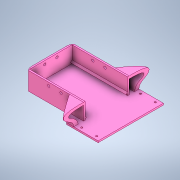
# Autodesk Inventor part: Body_001
Saved by Autodesk Inventor 2021 (Build 250183000, 183)
## iProperties
Created: 2022-04-07
Part Number: Body_001
Material: Genérico
Document SubType Name: Modeling
Designer: skatl
Density: 1 g/cm^3
Appearance: Rosado
Author: skatl
Autodesk Inventor part; units mm, degrees
ref_plane "YZ Plane" through (0, 0, 0) normal (1, 0, 0) x (0, 1, 0)
ref_plane "XZ Plane" through (0, 0, 0) normal (0, 1, 0) x (-1, 0, 0)
ref_plane "XY Plane" through (0, 0, 0) normal (0, 0, 1) x (1, 0, 0)
sketch "Boceto1" plane through (0, 0, 0) normal (0, 1, 0) x (-1, 0, 0)
  line L0 (-50, -35) -> (50, -35)
  line L1 (50, -35) -> (50, 35)
  line L2 (50, 35) -> (-50, 35)
  line L3 (-50, 35) -> (-50, -35)
  line L4 (-50, -35) -> (50, 35) construction
  line L5 (50, -35) -> (-50, 35) construction
  line L6 (-50, -35) -> (-20, -35)
  line L7 (-20, -35) -> (-20, 35)
  line L8 (-20, 35) -> (-50, 35)
  line L9 (-50, 35) -> (-50, -35)
  line L10 (-20, 40) -> (-50, 40)
  line L11 (-50, 40) -> (-50, -40)
  line L12 (-50, -40) -> (-20, -40)
  line L13 (-20, -40) -> (-20, 40)
  line L14 (-20, 40) -> (-50, -40) construction
  line L15 (-50, 40) -> (-20, -40) construction
  point P0 (0, 0)
  point P1 (-35, 0)
  dimension "d0" = 100
  dimension "d1" = 70
  dimension "d67" = 30
  dimension "d68" = 30
  dimension "d69" = 80
  constraints: 32 end point, 6 parallel, 4 midpoint, 3 horizontal, 3 perpendicular, 1 point on line
  measures "d0" distance of L2.end L1.end
  measures "d1" distance of L1.end L0.end
  measures "d67" distance of L8.end L7.end
  measures "d68" distance of L12.end L11.end
  measures "d69" distance of L11.end L10.end
extrude "Extrusión1" add sketch "Boceto1" along normal blind 22 contours L3 L2 L7 L0 | L7 L2 L1 L0
sketch "Boceto2" plane through (-50, 0, 35) normal (0, 0, 1) x (1, 0, 0)
  line L0 (0, 0) -> (100, 0) projected
  line L1 (100, 0) -> (70, 0)
  line L2 (70, 0) -> (70, 2)
  line L3 (70, 2) -> (100, 2)
  line L4 (100, 2) -> (100, 0)
  line L5 (0, 22) -> (100, 22) projected
  line L6 (70, 2) -> (100, 2)
  line L7 (100, 2) -> (100, 22)
  line L8 (100, 22) -> (70, 22)
  line L9 (70, 22) -> (70, 2)
  point P0 (50, 0)
  point P1 (70, 22)
  dimension "d4" = 30
  dimension "d5" = 2
  constraints: 16 end point, 4 parallel, 2 horizontal, 2 perpendicular
  measures "d4" distance of L2.end L3.end
  measures "d5" distance of L1.end L2.end
extrude "Extrusión2" cut sketch "Boceto2" against normal through all contours L9 L5 L7 L3
sketch "Boceto3" plane through (-50, 0, 35) normal (0, 0, 1) x (1, 0, 0)
  line L0 (70, 22) -> (0, 22) projected
  line L1 (35, 22) -> (35, 0)
  line L2 (70, 2) -> (70, 22) projected
  line L3 (70, 12) -> (-10, 12)
  line L4 (27.5, 3) -> (42.5, 3)
  line L5 (42.5, 3) -> (42.5, 21)
  line L6 (42.5, 21) -> (27.5, 21)
  line L7 (27.5, 21) -> (27.5, 3)
  line L8 (27.5, 3) -> (42.5, 21) construction
  line L9 (42.5, 3) -> (27.5, 21) construction
  line L10 (42.5, 21) -> (42.5, 18)
  circle A0 centre (42.5, 18) radius 1.5
  circle A1 centre (27.5, 18) radius 1.5
  point P0 (50, 0)
  point P1 (35, 12)
  dimension "d31" = 15
  dimension "d32" = 18
  dimension "d33" = 3
  dimension "d34" = 3
  constraints: 18 end point, 4 midpoint, 3 point on line, 2 centre point, 2 coincident, 2 horizontal, 2 parallel, 2 symmetric about line, 1 perpendicular, 1 vertical, 1 other
  measures "d31" distance of L6.end L5.end
  measures "d32" distance of L5.end L4.end
  measures "d33" distance of L5.end L10.end
  measures "d34" diameter of A0
extrude "Extrusión3" cut sketch "Boceto3" against normal through all contours A0 L5 | L5 A0 | A1 L7 | L7 A1
sketch "Boceto4" plane through (-50, 0, -35) normal (-1, 0, 0) x (0, 0, 1)
  line L0 (35, 22) -> (35, 0)
  line L1 (27.5, 3) -> (42.5, 3)
  line L2 (42.5, 3) -> (42.5, 21)
  line L3 (42.5, 21) -> (27.5, 21)
  line L4 (27.5, 21) -> (27.5, 3)
  line L5 (27.5, 3) -> (42.5, 21) construction
  line L6 (42.5, 3) -> (27.5, 21) construction
  line L7 (42.5, 21) -> (42.5, 18)
  circle A0 centre (42.5, 18) radius 1.5
  circle A1 centre (27.5, 18) radius 1.5
  line L8 (0, 22) -> (70, 22) projected
  line L9 (0, 22) -> (35, 22)
  line L10 (0, 0) -> (0, 22) projected
  point P0 (35, 0)
  point P1 (45, 0)
  point P2 (35, 12)
  point P3 (35, 12)
  dimension "d15" = 15
  dimension "d16" = 18
  dimension "d17" = 3
  dimension "d18" = 3
  dimension "d83" = 35
  constraints: 18 end point, 3 midpoint, 2 centre point, 2 parallel, 2 point on line, 1 coincident, 1 collinear, 1 horizontal, 1 perpendicular, 1 symmetric about line, 1 vertical, 1 other
  measures "d15" distance of L4.start L2.end
  measures "d16" distance of L2.end L2.start
  measures "d17" distance of L2.end L7.end
  measures "d18" diameter of A0
  measures "d83" distance between parallel lines of L10 L0
extrude "Extrusión4" cut sketch "Boceto4" against normal through all contours A0 L2 | L2 A0 | A1 L4 | L4 A1
sketch "Boceto5" plane through (20, 2, 35) normal (1, 0, 0) x (0, 0, -1)
  line L0 (0, 20) -> (70, 20) projected
  line L1 (35, 20) -> (61, 20)
  line L2 (61, 20) -> (61, 0)
  line L3 (0, 0) -> (70, 0) projected
  line L4 (35, 20) -> (9, 20)
  line L5 (9, 20) -> (9, 0)
  line L6 (9, 0) -> (61, 0)
  line L7 (61, 0) -> (61, 2)
  line L8 (61, 2) -> (59, 2)
  line L9 (59, 2) -> (61, 4)
  line L10 (9, 2) -> (11, 2)
  line L11 (11, 2) -> (9, 4)
  point P0 (35, -2)
  point P1 (9, 2)
  point P2 (9, 0)
  point P3 (9, 20)
  dimension "d21" = 26
  dimension "d22" = 26
  dimension "d23" = 2
  dimension "d24" = 2
  dimension "d25" = 45
  constraints: 20 end point, 5 point on line, 4 perpendicular, 1 midpoint
  measures "d21" distance of L1.start L1.end
  measures "d22" distance of L1.start L4.end
  measures "d23" distance of L2.end L7.end
  measures "d24" distance of L7.end L8.end
  measures "d25" angle of L8 L9
extrude "Extrusión5" cut sketch "Boceto5" against normal blind 68 contours L0 L2 L9 L8 L3 L5 L10 L11
sketch "Boceto6" plane through (0, 22, 0) normal (0, 1, 0) x (1, 0, 0)
  line L0 (-48, 26) -> (-48, -26) projected
  line L1 (-48, 26) -> (-16.5706, 52.8276)
  line L2 (-16.5706, 52.8276) -> (-58.9841, 16.6241)
  line L3 (-58.9841, 0) -> (-18.9783, 0)
  line L4 (-48, 26) -> (20, 26) projected
  line L5 (-48, 26) -> (-49.2985, 27.5212)
  line L6 (-49.2985, 27.5212) -> (-54.5232, 23.0614)
  line L7 (-54.5232, 23.0614) -> (-33.5838, 40.935)
  line L8 (-54.5232, 23.0614) -> (-54.5232, 44.2638)
  line L9 (-54.5232, 44.2638) -> (-32.2853, 44.2638)
  line L10 (-32.2853, 44.2638) -> (-33.5838, 40.935)
  line L11 (-48, -26) -> (-49.2985, -27.5212)
  line L12 (-49.2985, -27.5212) -> (-54.5232, -23.0614)
  line L13 (-54.5232, -23.0614) -> (-33.5838, -40.935)
  line L14 (-54.5232, -23.0614) -> (-54.5232, -44.2638)
  line L15 (-54.5232, -44.2638) -> (-32.2853, -44.2638)
  line L16 (-32.2853, -44.2638) -> (-33.5838, -40.935)
  point P0 (0, 0)
  dimension "d28" = 2
  constraints: 30 end point, 5 symmetric about line, 3 point on line, 2 perpendicular, 1 horizontal
  measures "d28" distance of L0.start L5.end
extrude "Extrusión6" cut sketch "Boceto6" against normal through all
fillet "Empalme1" radius 40 1 edges at (-40.5368, 11, 35)
fillet "Empalme2" radius 40 1 edges at (-40.5368, 11, -35)
fillet "Empalme3" radius 10 2 edges at (-50, 11, 26.9224) (-50, 11, -26.9224)
sketch "Boceto7" plane through (0, 22, 0) normal (0, 1, 0) x (1, 0, 0)
  line L0 (20, 26) -> (-48, 26) projected
  line L1 (20, 26) -> (20, 28)
  line L2 (20, 26) -> (20, 35) projected
  line L3 (20, 28) -> (-51.4254, 28)
  line L4 (-51.4254, 28) -> (-16.5183, 55.1765)
  line L5 (-16.5183, 55.1765) -> (20, 44.2601)
  line L6 (20, 44.2601) -> (20, 28)
  line L7 (22.0699, 0) -> (-59.6762, 0)
  line L8 (20, -28) -> (-51.4254, -28)
  line L9 (-51.4254, -28) -> (-16.5183, -55.1765)
  line L10 (-16.5183, -55.1765) -> (20, -44.2601)
  line L11 (20, -44.2601) -> (20, -28)
  point P0 (0, 0)
  point P1 (20, -35)
  dimension "d38" = 2
  constraints: 20 end point, 5 symmetric about line, 1 collinear, 1 horizontal, 1 perpendicular, 1 point on line
  measures "d38" distance of L0.start L1.end
extrude "Extrusión7" cut sketch "Boceto7" against normal up to surface (20 mm away)
sketch "Boceto8" plane through (50, 2, 35) normal (0, 1, 0) x (1, 0, 0)
  line L0 (-97.5807, 63) -> (-30, 63) projected
  line L1 (-30, 63) -> (-30, 70)
  line L2 (-75.8968, 70) -> (0, 70) projected
  line L3 (-64.3339, 63) -> (-30, 63)
  line L4 (-30, 61) -> (-98, 61) projected
  line L5 (-98, 61) -> (-98, 9) projected
  line L6 (-98, 35) -> (-56.2894, 35)
  line L7 (-30, 7) -> (-30, 0)
  line L8 (-30, 7) -> (-30, 9) projected
  line L9 (-30, 7) -> (-47.167, 7)
  line L10 (-97.5807, 7) -> (-30, 7) projected
  line L11 (0, 70) -> (0, 0) projected
  line L12 (0, 70) -> (-30, 70)
  line L13 (-30, 70) -> (-30, 0)
  line L14 (-30, 0) -> (0, 0)
  line L15 (0, 0) -> (0, 70)
  line L16 (-30, -5) -> (0, -5)
  line L17 (0, -5) -> (0, 75)
  line L18 (0, 75) -> (-30, 75)
  line L19 (-30, 75) -> (-30, -5)
  line L20 (-30, -5) -> (0, 75) construction
  line L21 (0, -5) -> (-30, 75) construction
  line L22 (-30, 75) -> (-47.167, 63)
  line L23 (-30, -5) -> (-47.167, 7)
  line L24 (-30, 61) -> (-30, 63) projected
  line L25 (-30, 63) -> (-30, 88)
  line L26 (-30, 88) -> (-47.167, 63)
  line L27 (-30, 7) -> (-30, -18)
  line L28 (-30, -18) -> (-47.167, 7)
  point P0 (-50, 35)
  point P1 (-15, 35)
  point P2 (-30, 0)
  point P3 (-30, 70)
  point P4 (-30, 75)
  point P5 (-30, -5)
  dimension "d57" = 30
  dimension "d58" = 80
  dimension "d74" = 25
  constraints: 42 end point, 5 parallel, 4 midpoint, 4 symmetric about line, 3 horizontal, 2 perpendicular, 2 point on line, 1 collinear, 1 vertical
  measures "d57" distance of L18.end L17.end
  measures "d58" distance of L17.end L16.end
  measures "d74" distance of L0.end L25.end
extrude "Extrusión8" add sketch "Boceto8" along normal blind 20 and the other way blind 2 contours L22 L2 L1 L0 | L26 L2 L22 | L22 L19 L2 | L2 L26 L25 L22 | L7 L19 L23 L9 | L23 L27 L28
sketch "Boceto13" plane through (20, 2, 35) normal (0, 1, 0) x (1, 0, 0)
  line L0 (0, 75) -> (30, 75)
  line L1 (30, 75) -> (30, -5)
  line L2 (30, -5) -> (0, -5)
  line L3 (0, -5) -> (0, 75)
  line L4 (0, 75) -> (30, -5) construction
  line L5 (30, 75) -> (0, -5) construction
  point P0 (-20, 35)
  point P1 (15, 35)
  dimension "d70" = 30
  dimension "d71" = 80
  constraints: 12 end point, 2 midpoint, 2 parallel, 1 horizontal, 1 perpendicular
  measures "d70" distance of L1.end L2.end
  measures "d71" distance of L0.end L1.end
extrude "Extrusión12" add sketch "Boceto13" against normal blind 2
sketch "Boceto14" plane through (-25.8968, 2, 35) normal (0, 1, 0) x (1, 0, 0)
  line L0 (-21.6839, 7) -> (28.7299, 7) projected
  line L1 (33.5366, 0) -> (28.7299, 7) projected
  line L2 (-21.6839, 7) -> (28.7299, 7)
  line L3 (28.7299, 7) -> (35.3305, -2.6123)
  line L4 (28.7299, 7) -> (45.8968, -18) projected
  line L5 (35.3305, -2.6123) -> (-21.6839, -2.6123)
  arc A0 (-24.1032, 13.5217) -> (-21.6839, 7) centre (-14.1032, 13.5217) ccw projected
  line L6 (-21.6839, -2.6123) -> (-21.6839, 7)
  line L7 (-21.6839, 7) -> (-33.4628, 7)
  line L8 (-33.4628, 7) -> (-34.2071, -2.6123)
  line L9 (-34.2071, -2.6123) -> (-21.6839, -2.6123)
  line L10 (-22.1032, 9) -> (-22.1032, 61) projected
  line L11 (-22.1032, 35) -> (32.0302, 35)
  line L12 (-21.6839, 63) -> (28.7299, 63)
  line L13 (33.5366, 70) -> (28.7299, 63)
  line L14 (-21.6839, 63) -> (28.7299, 63)
  line L15 (28.7299, 63) -> (35.3305, 72.6123)
  line L16 (35.3305, 72.6123) -> (-21.6839, 72.6123)
  arc A1 (-21.6839, 63) -> (-24.1032, 56.4783) centre (-14.1032, 56.4783) ccw
  line L17 (-21.6839, 72.6123) -> (-21.6839, 63)
  line L18 (-21.6839, 63) -> (-33.4628, 63)
  line L19 (-33.4628, 63) -> (-34.2071, 72.6123)
  line L20 (-34.2071, 72.6123) -> (-21.6839, 72.6123)
  point P0 (25.8968, 35)
  constraints: 34 end point, 9 symmetric about line, 5 point on line, 3 horizontal, 2 point on circle, 1 centre point, 1 collinear, 1 midpoint, 1 perpendicular, 1 other
extrude "Extrusión13" cut sketch "Boceto14" against normal through all
sketch "Boceto15" plane through (-50, 0, -21.4783) normal (-1, 0, 0) x (0, 0, 1)
  line L0 (21.4783, -4.1686) -> (21.4783, 27.0187)
  line L1 (42.9566, 22) -> (49.4783, 22) projected
  line L2 (49.4783, 22) -> (74.4783, 22)
  line L3 (74.4783, 22) -> (74.4783, 2)
  line L4 (74.4783, 2) -> (49.4783, 2)
  line L5 (49.4783, 2) -> (49.4783, 22)
  line L6 (49.4783, 22) -> (74.4783, 22) projected
  line L7 (49.4783, 22) -> (74.4783, 22) construction
  line L8 (74.4783, 22) -> (74.4783, 0) projected
  line L9 (74.4783, 22) -> (74.4783, 15.7481) construction
  line L10 (74.4783, 15.7481) -> (74.4783, 11) construction
  line L11 (74.4783, 11) -> (61.4783, 8.6537) construction
  line L12 (-18.5217, 2) -> (61.4783, 2) projected
  line L13 (61.4783, 8.6537) -> (61.4783, 2) construction
  spline S0 degree 4 poles (49.4783, 22) (74.4783, 22) (74.4783, 15.7481) (74.4783, 11) (61.4783, 8.6537) (61.4783, 2) knots 1 1 1 1 1 2 3 3 3 3 3
  line L14 (-4.5217, 2) -> (47.4783, 2) projected
  line L15 (21.4783, 2) -> (61.4783, 2)
  line L16 (49.4783, 22) -> (74.4783, 22) construction
  line L17 (74.4783, 22) -> (74.4783, 15.7481) construction
  line L18 (74.4783, 15.7481) -> (74.4783, 11) construction
  line L19 (74.4783, 11) -> (61.4783, 8.6537) construction
  line L20 (61.4783, 8.6537) -> (61.4783, 2) construction
  spline S1 degree 4 poles (49.4783, 22) (74.4783, 22) (74.4783, 15.7481) (74.4783, 11) (61.4783, 8.6537) (61.4783, 2) knots 1 1 1 1 1 2 3 3 3 3 3
  line L21 (49.4783, 18.8291) -> (68.2228, 18.8291) construction
  line L22 (68.2228, 18.8291) -> (68.2228, 14.1715) construction
  line L23 (68.2228, 14.1715) -> (67.7666, 11) construction
  line L24 (67.7666, 11) -> (58.5378, 11) construction
  line L25 (58.5378, 11) -> (55.8429, 2) construction
  spline S2 degree 4 poles (49.4783, 18.8291) (68.2228, 18.8291) (68.2228, 14.1715) (67.7666, 11) (58.5378, 11) (55.8429, 2) knots 1 1 1 1 1 2 3 3 3 3 3
  line L26 (-6.5217, 22) -> (-31.5217, 22)
  line L27 (-31.5217, 22) -> (-31.5217, 2)
  line L28 (-31.5217, 2) -> (-6.5217, 2)
  line L29 (-6.5217, 2) -> (-6.5217, 22)
  line L30 (-6.5217, 22) -> (-31.5217, 22)
  line L31 (-6.5217, 22) -> (-31.5217, 22) construction
  line L32 (-31.5217, 22) -> (-31.5217, 0)
  line L33 (-31.5217, 22) -> (-31.5217, 15.7481) construction
  line L34 (-31.5217, 15.7481) -> (-31.5217, 11) construction
  line L35 (-31.5217, 11) -> (-18.5217, 8.6537) construction
  line L36 (-18.5217, 8.6537) -> (-18.5217, 2) construction
  spline S3 degree 4 poles (-6.5217, 22) (-31.5217, 22) (-31.5217, 15.7481) (-31.5217, 11) (-18.5217, 8.6537) (-18.5217, 2) knots 1 1 1 1 1 2 3 3 3 3 3
  spline S4 degree 4 poles (-6.5217, 22) (-31.5217, 22) (-31.5217, 15.7481) (-31.5217, 11) (-18.5217, 8.6537) (-18.5217, 2) knots 1 1 1 1 1 2 3 3 3 3 3
  line L37 (-6.5217, 22) -> (-31.5217, 22) construction
  line L38 (-31.5217, 22) -> (-31.5217, 15.7481) construction
  line L39 (-31.5217, 15.7481) -> (-31.5217, 11) construction
  line L40 (-31.5217, 11) -> (-18.5217, 8.6537) construction
  line L41 (-18.5217, 8.6537) -> (-18.5217, 2) construction
  spline S5 degree 4 poles (-6.5217, 18.8291) (-25.2662, 18.8291) (-25.2662, 14.1715) (-24.81, 11) (-15.5812, 11) (-12.8863, 2) knots 1 1 1 1 1 2 3 3 3 3 3
  line L42 (-6.5217, 18.8291) -> (-25.2662, 18.8291) construction
  line L43 (-25.2662, 18.8291) -> (-25.2662, 14.1715) construction
  line L44 (-25.2662, 14.1715) -> (-24.81, 11) construction
  line L45 (-24.81, 11) -> (-15.5812, 11) construction
  line L46 (-15.5812, 11) -> (-12.8863, 2) construction
  line L47 (61.4783, 2) -> (47.4783, 2) projected
  line L48 (61.4783, 0) -> (74.4783, 0) projected
  line L49 (61.4783, 2) -> (74.4783, 2)
  line L50 (74.4783, 2) -> (74.4783, 0)
  line L51 (74.4783, 0) -> (61.4783, 0)
  line L52 (61.4783, 0) -> (61.4783, 2)
  line L53 (-4.5217, 2) -> (-18.5217, 2) projected
  line L54 (-31.5217, 0) -> (-18.5217, 0) projected
  line L55 (-18.5217, 2) -> (-31.5217, 2)
  line L56 (-31.5217, 2) -> (-31.5217, 0)
  line L57 (-31.5217, 0) -> (-18.5217, 0)
  line L58 (-18.5217, 0) -> (-18.5217, 2)
  point P0 (21.4783, 0)
  point P1 (55.8429, 2)
  point P2 (-6.5219, 22)
  point P3 (-6.5217, 2)
  point P4 (-12.8863, 2)
  dimension "d77" = 20
  dimension "d78" = 40
  constraints: 40 end point, 22 symmetric about line, 7 equal length, 4 horizontal, 4 perpendicular, 4 point on line, 2 coincident, 2 midpoint, 1 vertical, 18 other
  measures "d77" distance of L2.end L3.end
  measures "d78" distance of L15.start L12.end
extrude "Extrusión14" cut sketch "Boceto15" against normal through all contours L2 L3 L4 S0 | S2 L4 L5 | L4 L8 L48 L52 | L58 L54 L32 L28 | L28 L27 L26 S3 | S5 L29 L12
sketch "Boceto18" plane through (-48, 2, -26) normal (0, 1, 0) x (1, 0, 0)
  line L0 (68, 8.3646) -> (68, 14) projected
  line L1 (98, 14) -> (98, -66) projected
  line L2 (68, 14) -> (98, 14)
  line L3 (98, 14) -> (98, -66)
  line L4 (98, -66) -> (68, -66)
  line L5 (68, -66) -> (68, 14)
  line L6 (59.0732, 14) -> (98, 14) projected
  line L7 (83, 14) -> (83, 10)
  line L8 (83, 14) -> (87, 14) construction
  line L9 (83, 10) -> (73.9, 10)
  line L10 (83, 10) -> (92.1, 10)
  circle A0 centre (73.9, 10) radius 1.1
  circle A1 centre (92.1, 10) radius 1.1
  line L11 (66.892, -26) -> (102.7084, -26)
  circle A2 centre (73.9, -62) radius 1.1
  circle A3 centre (92.1, -62) radius 1.1
  dimension "d84" = 4
  dimension "d85" = 270
  dimension "d86" = 9.1
  dimension "d87" = 9.1
  dimension "d88" = 2.2
  dimension "d89" = 2.2
  constraints: 18 end point, 5 horizontal, 4 centre point, 2 coincident, 2 parallel, 2 perpendicular, 2 symmetric about line, 1 point on line, 1 vertical, 2 other
  measures "d84" distance of L7.start L7.end
  measures "d86" distance of L7.end L9.end
  measures "d87" distance of L7.end L10.end
  measures "d88" diameter of A0
  measures "d89" diameter of A1
extrude "Extrusión15" cut sketch "Boceto18" against normal through all contours A0 | A1 | A2 | A3
